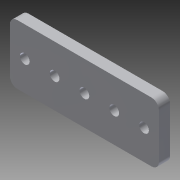
# Autodesk Inventor part: armbackspacer
Saved by Autodesk Inventor 2014 SP1 (Build 180222100, 222)
## iProperties
Created: 2014-01-05
Part Number: armbackspacer
Material: Aluminum 6061
Document SubType Name: Modeling
Designer: Arpan
Density: 2.71 g/cm^3
Appearance: Aluminum - Flat
Mass: 19.8362 g
Surface Area: 42.044 cm^2
Volume: 7.31964 cm^3
Author: Arpan
Autodesk Inventor part; units mm, degrees
ref_plane "YZ Plane" through (0, 0, 0) normal (1, 0, 0) x (0, 1, 0)
ref_plane "XZ Plane" through (0, 0, 0) normal (0, 1, 0) x (-1, 0, 0)
ref_plane "XY Plane" through (0, 0, 0) normal (0, 0, 1) x (1, 0, 0)
sketch "Sketch1" plane through (0, 0, 0) normal (0, 0, 1) x (1, 0, 0)
  line L0 (61.341, -25.4) -> (61.341, -2.159)
  line L1 (59.182, 0) -> (0, 0)
  line L2 (-2.159, -2.159) -> (-2.159, -25.4)
  circle A0 centre (29.591, -12.7) radius 2.0701
  circle A1 centre (54.991, -12.7) radius 2.0701
  circle A2 centre (4.191, -12.7) radius 2.0701
  circle A3 centre (16.891, -12.7) radius 2.0701
  circle A4 centre (42.291, -12.7) radius 2.0701
  line L3 (61.341, -25.4) -> (-2.159, -25.4)
  line L4 (-2.159, -25.4) -> (-2.159, 0)
  line L5 (-2.159, 0) -> (61.341, 0)
  line L6 (61.341, 0) -> (61.341, -25.4)
  dimension "d0" = 4.1402
  dimension "d1" = 90
  dimension "d2" = 63.5
  dimension "d3" = 0
  dimension "d4" = 25.4
  dimension "d5" = 61.341
  dimension "d6" = 0
  dimension "d7" = 2.159
  dimension "d8" = 2.159
  dimension "d9" = 6.35
  dimension "d10" = 12.7
  dimension "d11" = 19.05
  dimension "d12" = 12.7
  dimension "d13" = 31.75
  dimension "d14" = 12.7
  dimension "d15" = 44.45
  dimension "d16" = 12.7
  dimension "d17" = 57.15
  dimension "d18" = 12.7
  dimension "d19" = 61.341
  dimension "d20" = 2.159
  dimension "d21" = 25.4
  constraints: 14 end point, 5 centre point, 4 equal radius, 4 parallel, 1 horizontal, 1 perpendicular, 1 point on line
  measures "d0" diameter of A1
  measures "d1" angle of L1 L2
  measures "d2" distance between parallel lines of L6 L4
  measures "d3" distance between parallel lines of L1 L5
  measures "d4" distance between parallel lines of L1 L3
  measures "d5" distance from line of point (0, 0) L6
  measures "d6" distance from line of point (0, 0) L1
  measures "d7" distance from line of L0.end L1
  measures "d8" distance from line of L1.start L6
  measures "d9" distance from line of A1.centre L6
  measures "d10" distance from line of A1.centre L1
  measures "d11" distance from line of A4.centre L6
  measures "d12" distance from line of A4.centre L1
  measures "d13" distance from line of A0.centre L6
  measures "d14" distance from line of A0.centre L1
  measures "d15" distance from line of A3.centre L6
  measures "d16" distance from line of A3.centre L1
  measures "d17" distance from line of A2.centre L6
  measures "d18" distance from line of A2.centre L1
  measures "d19" distance from line of L1.end L6
  measures "d20" distance from line of L2.start L1
  measures "d21" distance from line of L2.end L1
extrude "Extrusion1" add sketch "Sketch1" along normal blind 4.7625
fillet "Fillet1" radius 3.175 4 edges at (61.341, 0, 2.3813) (-2.159, 0, 2.3813) (-2.159, -25.4, 2.3813) (61.341, -25.4, 2.3813)
body "Solid1"
